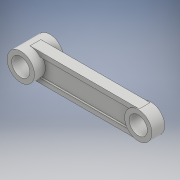
# Autodesk Inventor part: connecting_link
Saved by Autodesk Inventor 2018 (Build 220112000, 112)
## iProperties
Created: 2018-11-06
Part Number: connecting_link
Material: Generic
Document SubType Name: Modeling
Designer: HP
Density: 1 g/cm^3
Appearance: Default
Author: HP
Autodesk Inventor part; units mm, degrees
ref_plane "YZ Plane" through (0, 0, 0) normal (1, 0, 0) x (0, 1, 0)
ref_plane "XZ Plane" through (0, 0, 0) normal (0, 1, 0) x (-1, 0, 0)
ref_plane "XY Plane" through (0, 0, 0) normal (0, 0, 1) x (1, 0, 0)
sketch "Sketch1" plane through (0, 0, 0) normal (0, 1, 0) x (-1, 0, 0)
  line L0 (-60, -15) -> (60, -15)
  line L1 (60, -15) -> (60, 15)
  line L2 (60, 15) -> (-60, 15)
  line L3 (-60, 15) -> (-60, -15)
  line L4 (-60, -15) -> (60, 15) construction
  line L5 (60, -15) -> (-60, 15) construction
  circle A0 centre (-60, 0) radius 15
  circle A1 centre (60, 0) radius 15
  point P0 (0, 0)
  dimension "d0" = 120
  dimension "d1" = 30
  constraints: 12 end point, 4 midpoint, 2 parallel, 2 vertical alignment, 1 horizontal, 1 perpendicular, 4 other
  measures "d0" distance of L2.end L1.end
  measures "d1" distance of L1.end L0.end
extrude "Extrusion1" add sketch "Sketch1" along normal mid plane 12
sketch "Sketch2" plane through (0, 6, 0) normal (0, 1, 0) x (1, 0, 0)
  point P0 (0, 0)
sketch "Sketch3" plane through (0, 0, 0) normal (0, 1, 0) x (-1, 0, 0)
  circle A0 centre (60, 0) radius 15
  circle A1 centre (60, 0) radius 10
  point P0 (0, 0)
  dimension "d4" = 20
  constraints: 2 centre point, 1 coincident
  measures "d4" diameter of A1
extrude "Extrusion2" add sketch "Sketch3" along normal mid plane 32
sketch "Sketch4" plane through (0, 0, 0) normal (0, 1, 0) x (-1, 0, 0)
  circle A0 centre (-60, 0) radius 15
  circle A1 centre (-60, 0) radius 10
  point P0 (0, 0)
  dimension "d7" = 20
  constraints: 2 centre point, 1 coincident
  measures "d7" diameter of A1
extrude "Extrusion3" add sketch "Sketch4" along normal mid plane 14
sketch "Sketch5" plane through (0, 0, 0) normal (0, 1, 0) x (-1, 0, 0)
  point P0 (0, 0)
hole "Hole1" at (-60, 6, 0) direction (0, -1, 0) diameter 20 end through all
hole "Hole2" at (60, 6, 0) direction (0, -1, 0) diameter 20 end through all
sketch "Sketch6" plane through (0, 6, 0) normal (0, 1, 0) x (1, 0, 0)
  arc A0 (-48.8197, -10) -> (-48.8197, 10) centre (-60, 0) ccw
  arc A1 (48.8197, 10) -> (48.8197, -10) centre (60, 0) ccw
  circle A2 centre (-60, 0) radius 10 projected
  line L0 (48.8197, 10) -> (-48.8197, 10)
  line L1 (-60, 10) -> (-60, -10)
  line L2 (-48.8197, -10) -> (48.8197, -10)
  line L3 (60, -10) -> (60, 10)
  line L4 (60, 10) -> (-60, -10) construction
  line L5 (-60, 10) -> (60, -10) construction
  point P0 (0, 0)
  dimension "d28" = 30
  constraints: 12 end point, 4 point on circle, 2 centre point, 2 midpoint, 2 parallel, 1 horizontal, 1 perpendicular, 1 vertical alignment, 1 other
  measures "d28" diameter of A1
extrude "Extrusion4" cut sketch "Sketch6" against normal blind 2 contours A0 L0 A1 L2
mirror "Mirror1" about plane through (0, 0, 0) normal (0, 1, 0) of "Extrusion4"
body "Solid1"
